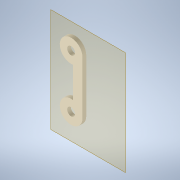
# Autodesk Inventor part: Encoder_Mount3_Washer
Saved by Autodesk Inventor 2022 (Build 260153000, 153)
## iProperties
Created: 2024-05-02
Part Number: Encoder_Mount3_Washer
Material: Generic
Document SubType Name: Modeling
Designer: Gotham City
Density: 1 g/cm^3
Appearance: Default
Author: Gotham City
Autodesk Inventor part; units mm, degrees
ref_plane "YZ Plane" through (0, 0, 0) normal (1, 0, 0) x (0, 1, 0)
ref_plane "XZ Plane" through (0, 0, 0) normal (0, 1, 0) x (-1, 0, 0)
ref_plane "XY Plane" through (0, 0, 0) normal (0, 0, 1) x (1, 0, 0)
ref_plane "Work Plane1" through (0, -5, 0) normal (0, 0, 1) x (-1, 0, 0)
sketch "Sketch1" plane through (0, -5, 0) normal (0, 0, 1) x (-1, 0, 0)
  circle A0 centre (3.5, 7) radius 1.05 projected
  circle A1 centre (3.5, 7) radius 3
  line L0 (-13.6, 0) -> (11.6, 0)
  circle A2 centre (3.5, -7) radius 1.05
  circle A3 centre (3.5, -7) radius 3
  line L1 (0.5, 7) -> (0.5, -7)
  line L2 (3.5, 7) -> (0.5, 7) construction
  line L3 (3, 4.042) -> (3, -4.042)
  point P0 (0, -5)
  dimension "d0" = 6
  dimension "d3" = 2.5
  constraints: 8 end point, 4 point on circle, 3 centre point, 2 coincident, 2 horizontal, 2 symmetric about line, 2 vertical, 4 other
  measures "d0" diameter of A1
  measures "d3" distance between parallel lines of L1 L3
extrude "Extrusion1" add sketch "Sketch1" against normal blind 1
body "Solid1"
